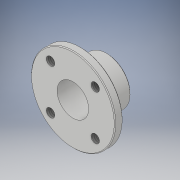
# Autodesk Inventor part: kolnierz
Saved by Autodesk Inventor 2019 (Build 230136000, 136)
## iProperties
Created: 2020-05-17
Part Number: kolnierz
Material: Generic
Document SubType Name: Modeling
Designer: estee
Density: 1 g/cm^3
Appearance: Default
Author: estee
Autodesk Inventor part; units mm, degrees
ref_plane "XY Plane" through (0, 0, 0) normal (0, 0, 1) x (1, 0, 0)
sketch "Sketch1" plane through (0, 0, 0) normal (1, 0, 0) x (0, 1, 0)
  line L0 (6, 0) -> (16, 0)
  line L1 (16, 0) -> (16, -3)
  line L2 (16, -3) -> (9, -3)
  line L3 (9, -3) -> (9, -13)
  line L4 (9, -13) -> (6, -13)
  line L5 (6, 0) -> (6, -13)
  line L6 (0, -15.6) -> (0, 2.6) projected
  point P0 (0, 0)
  dimension "d1" = 3
  dimension "d3" = 10
  dimension "d23" = 3
  dimension "d24" = 10
  dimension "d25" = 6
  constraints: 12 end point, 4 perpendicular, 1 horizontal
  measures "d1" distance of L0.end L1.end
  measures "d3" distance of L2.end L3.end
  measures "d23" distance between parallel lines of L3 L5
  measures "d24" distance of L0.start L0.end
  measures "d25" distance between parallel lines of L6 L5
revolve "Revolution1" add sketch "Sketch1" angle 360 about axis through (0, 0, -10) along (0, 0, 1)
chamfer "Chamfer1" distance 0.3 angle 45 3 edges at (0, -16, 0) (0, -16, -3) (0, -9, -13)
sketch "Sketch4" plane through (0, 0, 0) normal (0, 0, 1) x (1, 0, 0)
  line L0 (8.4853, 8.4853) -> (0, 0)
  line L1 (-22.4, 0) -> (22.4, 0) projected
  point P0 (8.4853, 8.4853)
  dimension "d37" = 45
  dimension "d38" = 8.4853
  constraints: 2 end point, 1 coincident
  measures "d37" angle of L1 L0
  measures "d38" horizontal distance of L0.end L0.start
hole "Hole3" at (8.4853, 8.4853, 0) direction (0, 0, -1) diameter 3.242 depth 6 tip angle 118 thread size "M4x0.7" class "6H" standard "ISO Metric profile"
pattern_circular "Circular Pattern1" count 4 over 360 about axis through (0, 0, -10) along (0, 0, 1) of "Hole3"
ref_plane "Work Plane1" through (0, 9, 0) normal (0, 1, 0) x (-1, 0, 0)
ref_plane "Work Plane2" through (9, 0, 0) normal (1, 0, 0) x (0, 1, 0)
sketch "Sketch5" plane through (0, 9, 0) normal (0, 1, 0) x (-1, 0, 0)
  line L0 (8.7, -13) -> (-8.7, -13) projected
  point P0 (0, 0)
  point P1 (0, -7)
  dimension "d41" = 6
  measures "d41" distance from line of L0 point (0, -7)
sketch "Sketch6" plane through (9, 0, 0) normal (1, 0, 0) x (0, 1, 0)
  line L0 (8.7, -13) -> (-8.7, -13) projected
  point P0 (0, 0)
  point P1 (0, -7)
  dimension "d42" = 6
  measures "d42" distance from line of L0 point (0, -7)
hole "Hole4" at (0, 9, -7) direction (0, -1, 0) diameter 2.459 depth 8.8 tip angle 118 thread size "M3x0.5" class "6H" standard "ISO Metric profile"
hole "Hole5" at (9, 0, -7) direction (-1, 0, 0) diameter 2.459 depth 8.8 tip angle 118 thread size "M3x0.5" class "6H" standard "ISO Metric profile"
body "Solid1"
